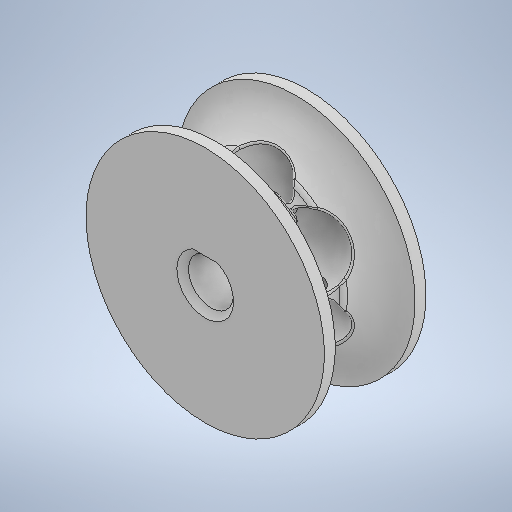
# Autodesk Inventor part: rope_shkif
Saved by Autodesk Inventor 2025.2 (Build 292293000, 293)
## iProperties
Created: 2025-01-25
Part Number: rope_shkif
Material: Типовые
Document SubType Name: Modeling
Designer: ignat
Density: 1 g/cm^3
Appearance: По умолчанию
Author: ignat
Autodesk Inventor part; units mm, degrees
ref_plane "YZ Plane" through (0, 0, 0) normal (1, 0, 0) x (0, 1, 0)
ref_plane "XZ Plane" through (0, 0, 0) normal (0, 1, 0) x (-1, 0, 0)
sketch "Эскиз1" plane through (0, 0, 0) normal (1, 0, 0) x (0, 1, 0)
  line L0 (0, 0) -> (8.2045, 0)
  line L1 (8.2045, 7) -> (0, 7)
  line L2 (0, 7) -> (0, 0)
  line L3 (8.2045, 0) -> (8.2045, 0.75)
  line L4 (8.2045, 6.25) -> (8.2045, 7)
  arc A0 (5.5, 3.9979) -> (5.5, 3.0021) centre (5.4545, 3.5) ccw
  arc A1 (8.2045, 6.25) -> (5.5, 3.9979) centre (8.2045, 3.5) ccw
  arc A2 (5.5, 3.0021) -> (8.2045, 0.75) centre (8.2045, 3.5) ccw
  line L5 (4.2955, 10.0695) -> (0, 10.0695)
  line L6 (0, 10.0695) -> (0, 12.5709)
  line L7 (0, 12.5709) -> (5.5, 12.5709)
  line L8 (4.2955, 8.9677) -> (5.5, 8.9677)
  dimension "d1" = 7
  dimension "d3" = 1
  dimension "d9" = 2.75
  dimension "d10" = 2.75
  dimension "d11" = 3.5
  dimension "d33" = 5.5
  constraints: 18 end point, 7 perpendicular, 6 point on circle, 3 centre point, 3 horizontal
  measures "d1" distance of L0.end L1.start
  measures "d3" diameter of A0
  measures "d9" radius of A1
  measures "d10" radius of A2
  measures "d11" distance from line of L0 A1.centre
  measures "d33" distance of L6.end L7.end
revolve "Вращение1" add sketch "Эскиз1" angle 360 about axis through (0, 0, 7) along (0, 0, -1)
sketch "Эскиз2" plane through (0, 0, 7) normal (0, 0, 1) x (1, 0, 0)
  arc A0 (-0.7616, 1.35) -> (0.7616, 1.35) centre (0, 0) ccw
  line L0 (-0.7616, 1.35) -> (0.7616, 1.35)
  dimension "d5" = 3.1
  constraints: 2 end point, 2 point on circle, 1 centre point, 1 coincident
  measures "d5" diameter of A0
extrude "Выдавливание1" cut sketch "Эскиз2" against normal through all
fillet "Сопряжение1" radius 0.4 2 edges at (0, -5.5, 3.9979) (0, -5.5, 3.0021)
ref_plane "РабПлоскость1" through (0, 0, 3.5) normal (0, 0, 1) x (1, 0, 0)
sketch "Эскиз3" plane through (0, 0, 3.5) normal (0, 0, 1) x (1, 0, 0)
  arc A0 (0, 6.2434) -> (0, 1.7434) centre (0, 3.9934) ccw
  circle A1 centre (45.9958, -0.3039) radius 5.5
  circle A2 centre (39.9958, -0.3039) radius 2.35
  circle A3 centre (43.2458, 4.4593) radius 2.35
  circle A4 centre (48.7458, 4.4593) radius 2.35
  circle A5 centre (51.4958, -0.3039) radius 2.35
  circle A6 centre (48.7458, -5.067) radius 2.35
  circle A7 centre (42.9958, -5.5) radius 2.35
  line L0 (0, 6.2434) -> (0, 1.7434)
  point P0 (0, 0)
  dimension "d13" = 4.5
  dimension "d16" = 11
  dimension "d19" = 4.7
  dimension "d20" = 4.7
  dimension "d21" = 4.7
  dimension "d22" = 4.7
  dimension "d23" = 4.7
  dimension "d24" = 4.7
  constraints: 8 centre point, 6 point on circle, 2 end point, 1 vertical
  measures "d13" diameter of A0
  measures "d16" diameter of A1
  measures "d19" diameter of A2
  measures "d20" diameter of A3
  measures "d21" diameter of A4
  measures "d22" diameter of A5
  measures "d23" diameter of A6
  measures "d24" diameter of A7
revolve "Вращение2" cut sketch "Эскиз3" angle 360 about axis through (0, 6.2434, 3.5) along (0, -1, 0) contours L0 A0
pattern_circular "Круговой массив1" count 6 over 360 about axis through (0, 0, 7) along (0, 0, -1) of "Вращение2"
fillet "Сопряжение2" radius 0.1 44 edges at (-1.8479, 5.1396, 4.0781) (1.8479, 5.1396, 4.0781) (2.206, 4.4363, 3.5) (1.8479, 5.1396, 2.9219) (-1.8479, 5.1396, 2.9219) (0.9036, 5.6626, 2.2917) (-0.9036, 5.6626, 2.2917) (0.9036, 5.6626, 4.7083) (-0.9036, 5.6626, 4.7083) (3.5271, -4.1701, 2.9219) (5.3749, -0.9695, 2.9219) (2.739, -4.1286, 3.5) (3.5271, -4.1701, 4.0781) (5.3749, -0.9695, 4.0781) (5.0248, -2.9011, 4.8383) (5.0248, -2.9011, 2.1617) (-5.3749, -0.9695, 2.9219) (-3.5271, -4.1701, 2.9219) (-4.945, -0.3077, 3.5) (-5.3749, -0.9695, 4.0781) (-3.5271, -4.1701, 4.0781) (-5.0248, -2.9011, 4.8383) (-5.0248, -2.9011, 2.1617) (-3.5271, 4.1701, 2.9219) (-5.3749, 0.9695, 2.9219) (-2.739, 4.1286, 3.5) (-3.5271, 4.1701, 4.0781) (-5.3749, 0.9695, 4.0781) (-5.0248, 2.9011, 4.8383) (-5.0248, 2.9011, 2.1617) (5.3749, 0.9695, 2.9219) (3.5271, 4.1701, 2.9219) (4.945, 0.3077, 3.5) (5.3749, 0.9695, 4.0781) (3.5271, 4.1701, 4.0781) (5.0248, 2.9011, 4.8383) (5.0248, 2.9011, 2.1617) (-1.8479, -5.1396, 2.9219) (1.8479, -5.1396, 2.9219) (-2.206, -4.4363, 3.5) (-1.8479, -5.1396, 4.0781) (1.8479, -5.1396, 4.0781) (0, -5.8022, 4.8383) (0, -5.8022, 2.1617)
chamfer "Фаска1" distance 0.4 angle 45 4 edges at (0, 1.35, 7) (0, -1.55, 7) (0, -1.55, 0) (0, 1.35, 0)
